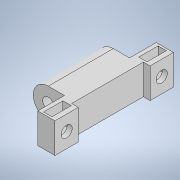
# Autodesk Inventor part: Крепление Open MV
Saved by Autodesk Inventor 2020 (Build 240168000, 168)
## iProperties
Created: 2019-06-16
Part Number: Крепление Open MV
Material: Типовые
Document SubType Name: Modeling
Designer: ivanc
Density: 1 g/cm^3
Appearance: По умолчанию
Author: ivanc
Autodesk Inventor part; units mm, degrees
ref_plane "YZ Plane" through (0, 0, 0) normal (1, 0, 0) x (0, 1, 0)
ref_plane "XZ Plane" through (0, 0, 0) normal (0, 1, 0) x (-1, 0, 0)
ref_plane "XY Plane" through (0, 0, 0) normal (0, 0, 1) x (1, 0, 0)
sketch "Эскиз1" plane through (0, 0, 0) normal (0, 0, 1) x (1, 0, 0)
  line L0 (0, 0) -> (8, 0)
  line L1 (8, 0) -> (8, 9)
  line L2 (8, 9) -> (0, 9)
  line L3 (0, 9) -> (0, 0)
  circle A0 centre (0, 4.5) radius 4.5
  dimension "d0" = 8
  dimension "d1" = 9
  constraints: 8 end point, 2 parallel, 1 horizontal, 1 midpoint, 1 perpendicular, 3 other
  measures "d0" distance of L2.end L1.end
  measures "d1" distance of L1.end L0.end
extrude "Выдавливание1" add sketch "Эскиз1" along normal blind 35.5
sketch "Эскиз2" plane through (8, 0, 0) normal (1, 0, 0) x (0, 0, -1)
  line L0 (-35.5, 0) -> (-35.5, 9) projected
  line L1 (0, 0) -> (-35.5, 0) projected
  line L2 (-35.5, 9) -> (-28.5, 9)
  line L3 (-28.5, 9) -> (-28.5, 0)
  line L4 (-28.5, 0) -> (-35.5, 0)
  line L5 (-35.5, 0) -> (-35.5, 9)
  line L6 (0, 0) -> (0, 9) projected
  line L7 (0, 9) -> (-7, 9)
  line L8 (-7, 9) -> (-7, 0)
  line L9 (-7, 0) -> (0, 0)
  line L10 (0, 0) -> (0, 9)
  dimension "d4" = 7
  dimension "d5" = 7
  constraints: 16 end point, 4 parallel, 2 horizontal, 2 perpendicular, 2 point on line
  measures "d4" distance of L3.end L4.end
  measures "d5" distance of L9.end L8.end
extrude "Выдавливание2" add sketch "Эскиз2" along normal blind 2
sketch "Эскиз3" plane through (10, 0, 0) normal (1, 0, 0) x (0, 0, -1)
  line L0 (-35.5, 9) -> (-35.5, 0) projected
  line L1 (-35.5, 4.5) -> (-28.5, 4.5)
  line L2 (-28.5, 0) -> (-28.5, 9) projected
  line L3 (-7, 9) -> (-7, 0) projected
  line L4 (-7, 4.5) -> (0, 4.5)
  line L5 (0, 9) -> (0, 0) projected
  point P0 (-32, 4.5)
  point P1 (-3.5, 4.5)
  constraints: 6 midpoint, 4 end point
hole "Отверстие1" at (10, 4.5, 32) at (10, 4.5, 3.5) direction (-1, 0, 0) diameter 3.35 depth 4
sketch "Эскиз4" plane through (10, 0, 0) normal (1, 0, 0) x (0, 0, -1)
  circle A0 centre (-32, 4.5) radius 1.675 projected
  line L0 (-34.9, 6.1743) -> (-32, 7.8486)
  line L1 (-32, 7.8486) -> (-29.1, 6.1743)
  line L2 (-29.1, 6.1743) -> (-29.1, 2.8257)
  line L3 (-29.1, 2.8257) -> (-32, 1.1514)
  line L4 (-32, 1.1514) -> (-34.9, 2.8257)
  line L5 (-34.9, 2.8257) -> (-34.9, 6.1743)
  circle A1 centre (-3.5, 4.5) radius 1.675 projected
  line L6 (-6.4, 6.1743) -> (-3.5, 7.8486)
  line L7 (-3.5, 7.8486) -> (-0.6, 6.1743)
  line L8 (-0.6, 6.1743) -> (-0.6, 2.8257)
  line L9 (-0.6, 2.8257) -> (-3.5, 1.1514)
  line L10 (-3.5, 1.1514) -> (-6.4, 2.8257)
  line L11 (-6.4, 2.8257) -> (-6.4, 6.1743)
  line L12 (0, 9) -> (-35.5, 9) projected
  line L13 (-6.4, 6.1743) -> (-0.6, 6.1743)
  line L14 (-0.6, 6.1743) -> (-0.6, 9)
  line L15 (-0.6, 9) -> (-6.4, 9)
  line L16 (-6.4, 9) -> (-6.4, 6.1743)
  line L17 (-29.1, 6.1743) -> (-34.9, 6.1743)
  line L18 (-34.9, 6.1743) -> (-34.9, 9)
  line L19 (-34.9, 9) -> (-29.1, 9)
  line L20 (-29.1, 9) -> (-29.1, 6.1743)
  point P0 (0, 0)
  dimension "d15" = 5.8
  dimension "d16" = 5.8
  constraints: 40 end point, 4 parallel, 2 coincident, 2 horizontal, 2 perpendicular, 2 point on line, 26 other
  measures "d15" distance between parallel lines of L8 L11
  measures "d16" distance between parallel lines of L2 L5
extrude "Выдавливание3" cut sketch "Эскиз4" along normal blind 2.5 from surface at -4
sketch "Эскиз5" plane through (0, 0, 35.5) normal (0, 0, 1) x (1, 0, 0)
  line L0 (0, 9) -> (10, 9) projected
  circle A0 centre (0, 4.5) radius 4.5
  arc A1 (0, 9) -> (0, 0) centre (0, 4.5) ccw projected
  line L1 (0, 9) -> (4.85, 9)
  line L2 (4.85, 9) -> (4.85, 0)
  line L3 (4.85, 0) -> (0, 0)
  line L4 (0, 0) -> (0, 9)
  point P0 (0, 0)
  dimension "d40" = 9
  dimension "d41" = 4.85
  constraints: 8 end point, 2 parallel, 1 coincident, 1 horizontal, 1 perpendicular, 2 other
  measures "d41" distance of L0.start L1.end
extrude "Выдавливание4" cut sketch "Эскиз5" against normal blind 8
sketch "Эскиз6" plane through (0, 0, 0) normal (0, 0, -1) x (-1, 0, 0)
  circle A0 centre (0, 4.5) radius 4.5
  line L0 (0, 9) -> (-10, 9) projected
  line L1 (0, 9) -> (-4.85, 9)
  line L2 (-4.85, 9) -> (-4.85, 0)
  line L3 (-4.85, 0) -> (0, 0)
  line L4 (0, 0) -> (0, 9)
  point P0 (0, 0)
  dimension "d42" = 9
  dimension "d43" = 4.85
  constraints: 8 end point, 2 parallel, 1 centre point, 1 coincident, 1 horizontal, 1 perpendicular
  measures "d42" diameter of A0
  measures "d43" distance of L2.end L3.end
extrude "Выдавливание5" cut sketch "Эскиз6" against normal blind 8
sketch "Эскиз7" plane through (0, 0, 8) normal (0, 0, -1) x (-1, 0, 0)
  arc A0 (0, 0) -> (0, 9) centre (0, 4.5) ccw projected
  constraints: 1 coincident
hole "Отверстие2" at (0, 4.5, 8) direction (0, 0, 1) diameter 3.35 end through all
equation "\"d16\" = d15"
